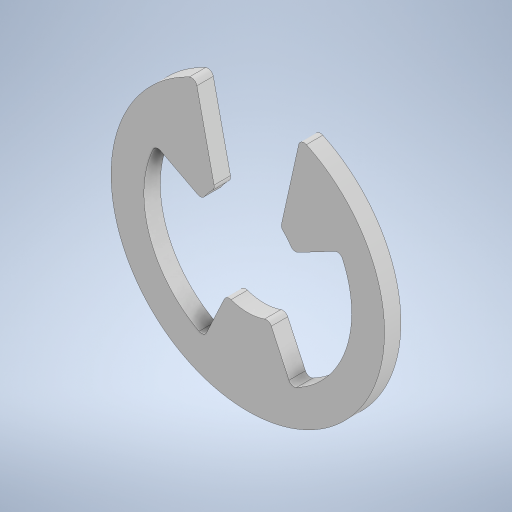
# Autodesk Inventor part: SA E-Clip
Saved by Autodesk Inventor 2024 (Build 280153000, 153)
## iProperties
Created: 2023-06-24
Part Number: SA E-Clip
Material: Generic
Document SubType Name: Modeling
Designer: birud
Density: 1 g/cm^3
Appearance: Default
Author: birud
Autodesk Inventor part; units mm, degrees
ref_plane "YZ Plane" through (0, 0, 0) normal (1, 0, 0) x (0, 1, 0)
ref_plane "XZ Plane" through (0, 0, 0) normal (0, 1, 0) x (-1, 0, 0)
ref_plane "XY Plane" through (0, 0, 0) normal (0, 0, 1) x (1, 0, 0)
sketch "Sketch1" plane through (0, 0, 0) normal (0, 0, 1) x (1, 0, 0)
  circle A0 centre (0, 0) radius 1.1906
  circle A1 centre (0, 0) radius 3.175
  dimension "d0" = 2.3813
  dimension "d1" = 6.35
  constraints: 2 centre point, 2 coincident
  measures "d0" diameter of A0
  measures "d1" diameter of A1
extrude "Extrusion1" add sketch "Sketch1" along normal mid plane 0.381
sketch "Sketch2" plane through (0, 0, 0.1905) normal (0, 0, 1) x (1, 0, 0)
  circle A0 centre (0, 0) radius 1.1906 projected
  circle A1 centre (0, 0) radius 3.175 projected
  line L0 (-0.635, 0.3107) -> (0.635, 0.3107)
  line L1 (0.635, 0.3107) -> (1.27, 3.175)
  line L2 (1.27, 3.175) -> (-1.27, 3.175)
  line L3 (-1.27, 3.175) -> (-0.635, 0.3107)
  circle A2 centre (0, 0) radius 1.1906 projected
  circle A3 centre (0, 0) radius 3.175 projected
  line L4 (0, 4.445) -> (0, -4.445) projected
  dimension "d4" = 1.27
  dimension "d5" = 2.54
  dimension "d6" = 25
  constraints: 8 end point, 1 horizontal, 1 parallel, 1 tangent, 1 other
  measures "d4" distance of L0.start L0.end
  measures "d5" distance of L1.end L2.end
  measures "d6" angle of L1 L3
extrude "Extrusion2" cut sketch "Sketch2" against normal blind 0.381 contours L1 L0 L4 A0 | A0 L4 A1 L1 | L4 L0 L3 A0 | A0 L3 A1 L4 | A1 L2 L1 | A1 L3 L2 picked at (0.3904, 0.5615) picked at (0.7715, 2.3859) picked at (-0.3904, 0.5615) picked at (-0.7715, 2.3859)
sketch "Sketch3" plane through (0, 0, 0.1905) normal (0, 0, 1) x (1, 0, 0)
  arc A0 (-1.2163, 2.9328) -> (1.2163, 2.9328) centre (0, 0) ccw projected
  arc A1 (-2.1409, 1.1132) -> (2.1409, 1.1132) centre (0, 0) ccw
  line L0 (-2.1409, 1.1132) -> (-1.0566, 0.5487)
  arc A2 (-0.7678, 0.9099) -> (0.7678, 0.9099) centre (0, 0) ccw projected
  line L1 (2.1409, 1.1132) -> (1.0566, 0.5487)
  line L2 (0, 4.1543) -> (0, -4.3966) projected
  line L3 (-0.7678, 0.9099) -> (-1.2163, 2.9328) projected
  line L4 (-0.4953, -1.0827) -> (-1.0119, -2.1906)
  line L5 (0.4953, -1.0827) -> (1.0119, -2.1906)
  dimension "d9" = 0.762
  dimension "d10" = 50
  dimension "d11" = 50
  dimension "d12" = 2.1133
  dimension "d13" = 0.9906
  constraints: 8 end point, 8 point on circle, 1 centre point, 2 other
  measures "d9" radial gap between concentric circles of A0 A1
  measures "d10" angle of L0 L3
  measures "d11" angle of L5 L4
  measures "d12" distance of L1.end L0.end
  measures "d13" distance of L5.start L4.start
extrude "Extrusion3" cut sketch "Sketch3" against normal blind 0.381 contours A2 L4 A1 L0 | L5 A2 L1 A1
fillet "Fillet1" radius 0.127 12 edges at (-1.2163, 2.9328, 0) (1.2163, 2.9328, 0) (-0.7678, 0.9099, 0) (-1.0566, 0.5487, 0) (0.7678, 0.9099, 0) (1.0566, 0.5487, 0) (2.1409, 1.1132, 0) (-2.1409, 1.1132, 0) (-1.0119, -2.1906, 0) (-0.4953, -1.0827, 0) (0.4953, -1.0827, 0) (1.0119, -2.1906, 0)
scale "Scale1" factors (10, 10, 10) then translate (0, 0, 1.7145) bodies 1
body "Solid1"
